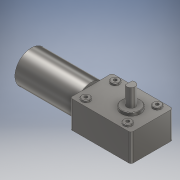
# Autodesk Inventor part: uxcell 12V 6RPM 6mm Worm Gear Motor
Saved by Autodesk Inventor 2017 SP1 (Build 210196100, 196)
## iProperties
Created: 2017-11-07
Part Number: uxcell 12V 6RPM 6mm Worm Gear Motor
Material: Stainless Steel
Document SubType Name: Modeling
Designer: Zach
Density: 8 g/cm^3
Appearance: Semi-Polished
Author: Zach
Autodesk Inventor part; units mm, degrees
ref_plane "YZ Plane" through (0, 0, 0) normal (1, 0, 0) x (0, 1, 0)
ref_plane "XZ Plane" through (0, 0, 0) normal (0, 1, 0) x (-1, 0, 0)
ref_plane "XY Plane" through (0, 0, 0) normal (0, 0, 1) x (1, 0, 0)
sketch "Sketch1" plane through (0, 0, 0) normal (0, 0, 1) x (1, 0, 0)
  line L0 (0, 0) -> (58, 0)
  line L1 (58, 0) -> (58, 40)
  line L2 (58, 40) -> (0, 40)
  line L3 (0, 40) -> (0, 0)
  line L4 (9, 34) -> (49, 34) construction
  line L5 (49, 34) -> (49, 6) construction
  line L6 (49, 6) -> (9, 6) construction
  line L7 (9, 6) -> (9, 34) construction
  circle A0 centre (49, 34) radius 1.5
  circle A1 centre (49, 6) radius 1.5
  circle A2 centre (9, 34) radius 1.5
  circle A3 centre (9, 6) radius 1.5
  point P0 (49, 20)
  point P1 (0, 20)
  point P2 (29, 34)
  point P3 (29, 40)
  dimension "d0" = 58
  dimension "d1" = 40
  dimension "d2" = 40
  dimension "d3" = 28
  dimension "d4" = 3
  dimension "d5" = 3
  dimension "d6" = 3
  dimension "d7" = 3
  constraints: 16 end point, 4 centre point, 4 coincident, 4 midpoint, 4 parallel, 2 horizontal, 2 perpendicular, 1 horizontal alignment, 1 vertical alignment
  measures "d0" distance of L2.end L1.end
  measures "d1" distance of L1.end L0.end
  measures "d2" distance of L5.end L6.end
  measures "d3" distance of L4.end L5.end
  measures "d4" diameter of A0
  measures "d5" diameter of A1
  measures "d6" diameter of A2
  measures "d7" diameter of A3
extrude "Extrusion1" add sketch "Sketch1" along normal blind 26
sketch "Sketch2" plane through (0, 0, 26) normal (0, 0, 1) x (1, 0, 0)
  circle A0 centre (38, 20) radius 4
  line L0 (58, 0) -> (58, 40) projected
  circle A1 centre (49, 34) radius 1.5 projected
  point P0 (0, 0)
  point P1 (58, 20)
  dimension "d10" = 8
  dimension "d12" = 11
  constraints: 1 centre point, 1 horizontal alignment, 1 midpoint
  measures "d10" diameter of A0
  measures "d12" horizontal distance of A1.centre A0.centre
extrude "Extrusion2" add sketch "Sketch2" along normal blind 20 contours A0
sketch "Sketch3" plane through (0, 0, 26) normal (0, 0, 1) x (1, 0, 0)
  circle A0 centre (38, 20) radius 4 projected
  circle A1 centre (38, 20) radius 9
  point P0 (0, 0)
  dimension "d15" = 18
  constraints: 1 centre point, 1 coincident
  measures "d15" diameter of A1
extrude "Extrusion3" add sketch "Sketch3" along normal blind 3
fillet "Fillet1" radius 2 4 edges at (58, 40, 13) (58, 0, 13) (0, 40, 13) (0, 0, 13)
sketch "Sketch4" plane through (0, 2, 0) normal (-1, 0, 0) x (0, 0, 1)
  circle A0 centre (13, 18) radius 15.5
  line L0 (0, 36) -> (0, 0) projected
  line L1 (26, 38) -> (0, 38) projected
  point P0 (0, -2)
  point P1 (0, 18)
  point P2 (13, 38)
  dimension "d19" = 31
  constraints: 2 midpoint, 1 centre point, 1 horizontal alignment, 1 vertical alignment
  measures "d19" diameter of A0
extrude "Extrusion4" add sketch "Sketch4" along normal blind 57
sketch "Sketch5" plane through (38, 20, 46) normal (0, 0, 1) x (1, 0, 0)
  circle A0 centre (0, 0) radius 4 construction
  line L0 (-2.2, 3.3407) -> (-2.2, -3.3407)
  arc A1 (-2.2, 3.3407) -> (-2.2, -3.3407) centre (0, 0) ccw
  point P0 (-38, -20)
  dimension "d22" = 2.2
  constraints: 4 point on circle, 2 end point, 1 centre point, 1 concentric, 1 vertical
  measures "d22" distance from line of A0.centre L0
extrude "Extrusion5" cut sketch "Sketch5" against normal blind 12
sketch "Sketch6" plane through (0, 0, 26) normal (0, 0, 1) x (1, 0, 0)
  circle A0 centre (49, 34) radius 1.5 projected
  circle A1 centre (49, 6) radius 1.5 projected
  circle A2 centre (9, 6) radius 1.5 projected
  circle A3 centre (9, 34) radius 1.5 projected
  circle A4 centre (9, 34) radius 4
  circle A5 centre (9, 6) radius 4
  circle A6 centre (49, 6) radius 4
  circle A7 centre (49, 34) radius 4
  point P0 (0, 0)
  dimension "d25" = 8
  dimension "d26" = 8
  dimension "d27" = 8
  dimension "d28" = 8
  constraints: 4 centre point, 4 coincident
  measures "d25" diameter of A4
  measures "d26" diameter of A5
  measures "d27" diameter of A6
  measures "d28" diameter of A7
extrude "Extrusion6" add sketch "Sketch6" along normal blind 2
sketch "Sketch8" plane through (0, 0, 0) normal (0, 0, -1) x (-1, 0, 0)
  circle A0 centre (-9, 6) radius 1.5 projected
  circle A1 centre (-9, 34) radius 1.5 projected
  circle A2 centre (-49, 6) radius 1.5 projected
  circle A3 centre (-49, 34) radius 1.5 projected
  arc A4 (-2, 0) -> (0, 2) centre (-2, 2) ccw construction
  line L0 (0, 38) -> (0, 28.441) construction
  arc A5 (0, 38) -> (-2, 40) centre (-2, 38) ccw construction
  line L1 (-56, 40) -> (-2, 40) construction
  arc A6 (-56, 40) -> (-58, 38) centre (-56, 38) ccw construction
  line L2 (-58, 2) -> (-58, 38) construction
  arc A7 (-58, 2) -> (-56, 0) centre (-56, 2) ccw construction
  line L3 (-2, 0) -> (-56, 0) construction
  line L4 (0, 11.559) -> (0, 2) projected
  line L5 (0, 28.441) -> (0, 11.559) projected
  point P0 (0, 0)
extrude "Extrusion7" add sketch "Sketch8" against normal blind 14
fillet "Fillet2" radius 0.5 5 edges at (45, 34, 28) (45, 6, 28) (5, 6, 28) (5, 34, 28) (29, 20, 29)
sketch "Sketch9" plane through (-57, 20, 13) normal (-1, 0, 0) x (0, 0, 1)
  line L0 (-1.5, 11) -> (1.5, 11)
  line L1 (1.5, 11) -> (1.5, 10.5)
  line L2 (1.5, 10.5) -> (-1.5, 10.5)
  line L3 (-1.5, 10.5) -> (-1.5, 11)
  line L4 (-1.5, -10.5) -> (1.5, -10.5)
  line L5 (1.5, -10.5) -> (1.5, -11)
  line L6 (1.5, -11) -> (-1.5, -11)
  line L7 (-1.5, -11) -> (-1.5, -10.5)
  circle A0 centre (0, 0) radius 15.5 construction
  point P0 (-13, -20)
  point P1 (0, 10.5)
  dimension "d34" = 3
  dimension "d35" = 0.5
  dimension "d36" = 3
  dimension "d37" = 0.5
  dimension "d38" = 10.5
  dimension "d39" = 10.5
  constraints: 16 end point, 4 parallel, 2 horizontal, 2 perpendicular, 1 midpoint, 1 point on line, 1 vertical alignment
  measures "d34" distance of L1.end L2.end
  measures "d35" distance of L0.end L1.end
  measures "d36" distance of L5.end L6.end
  measures "d37" distance of L4.end L5.end
  measures "d38" distance of A0.centre point (0, 10.5)
  measures "d39" distance from line of L4 A0.centre
extrude "Extrusion8" add sketch "Sketch9" along normal blind 3
sketch "Sketch10" plane through (-57, 30.5, 11.5) normal (0, -1, 0) x (1, 0, 0)
  circle A0 centre (-1.5, 1.5) radius 1.5 construction
  line L0 (0, 3) -> (-3, 3) construction
  line L1 (0, 0) -> (-3, 0) construction
  line L2 (-3, 3) -> (-3, 0) construction
  circle A1 centre (-1.5, 1.5) radius 0.5
  line L3 (-1.5, 0) -> (-3, 0)
  line L4 (-3, 0) -> (-3, 1.5)
  line L5 (-3, 1.5) -> (-3, 3)
  line L6 (-1.5, 3) -> (-3, 3)
  arc A2 (-1.5, 3) -> (-3, 1.5) centre (-1.5, 1.5) ccw
  arc A3 (-3, 1.5) -> (-1.5, 0) centre (-1.5, 1.5) ccw
  point P0 (57, -11.5)
  dimension "d43" = 1
  constraints: 8 end point, 8 tangent, 4 centre point, 4 point on circle, 3 collinear, 3 midpoint, 1 coincident, 1 concentric
  measures "d43" diameter of A1
extrude "Extrusion9" cut sketch "Sketch10" along normal through all both and the other way through all
sketch "Sketch11" plane through (-57, 20, 13) normal (-1, 0, 0) x (0, 0, 1)
  circle A0 centre (0, 0) radius 3
  circle A1 centre (0, 0) radius 15.5 construction
  point P0 (-13, -20)
  dimension "d46" = 6
  constraints: 1 centre point, 1 coincident
  measures "d46" diameter of A0
extrude "Extrusion10" add sketch "Sketch11" along normal blind 1
fillet "Fillet4" radius 0.5 1 edges at (-58, 20, 10)
body "Solid1"
